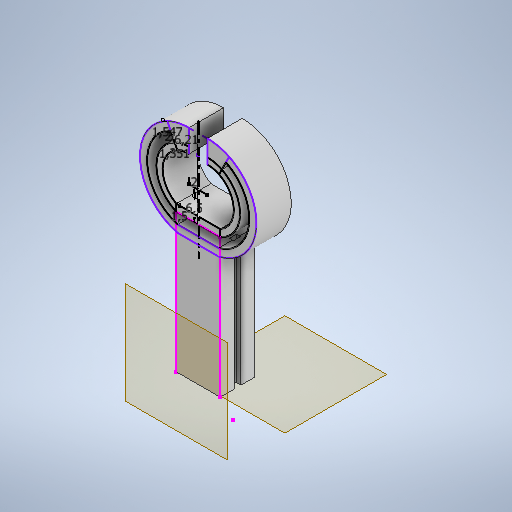
# Autodesk Inventor part: SlangHållare
Saved by Autodesk Inventor 2025.2 (Build 292293000, 293)
## iProperties
Created: 2025-01-28
Part Number: SlangHållare
Material: Generic
Document SubType Name: Modeling
Designer: 24oscnor
Density: 1 g/cm^3
Appearance: Default
Author: 24oscnor
Autodesk Inventor part; units mm, degrees
ref_plane "YZ Plane" through (0, 0, 0) normal (1, 0, 0) x (0, 1, 0)
ref_plane "XZ Plane" through (0, 0, 0) normal (0, 1, 0) x (-1, 0, 0)
ref_plane "XY Plane" through (0, 0, 0) normal (0, 0, 1) x (1, 0, 0)
ref_plane "Work Plane1" through (0, 3, 0) normal (0, 1, 0) x (1, 0, 0)
sketch "Sketch2" plane through (0, 3, 0) normal (0, 1, 0) x (1, 0, 0)
  line L0 (-11.25, -11.25) -> (-3.75, -11.25)
  line L1 (-3.75, -11.25) -> (-3.75, -3.75)
  line L2 (-3.75, -3.75) -> (-11.25, -3.75)
  line L3 (-11.25, -3.75) -> (-11.25, -11.25)
  line L4 (0, -15) -> (0, 0) projected
  line L5 (0, 0) -> (-15, 0) projected
  line L6 (-3.75, -11.25) -> (-2.75, -11.25)
  line L7 (-2.75, -11.25) -> (-2.75, -8.25)
  line L8 (-2.75, -8.25) -> (-3.75, -8.25)
  line L9 (-3.75, -8.25) -> (-3.75, -11.25)
  line L10 (-14.1659, -7.5) -> (-0.7229, -7.5) construction
  line L11 (-7.5, -11.25) -> (-7.5, -3.75) construction
  line L12 (-3.75, -3.75) -> (-2.75, -3.75)
  line L13 (-2.75, -3.75) -> (-2.75, -6.75)
  line L14 (-2.75, -6.75) -> (-3.75, -6.75)
  line L15 (-11.25, -11.25) -> (-12.25, -11.25)
  line L16 (-12.25, -11.25) -> (-12.25, -8.25)
  line L17 (-12.25, -8.25) -> (-11.25, -8.25)
  line L18 (-0.8341, -7.5) -> (-14.2771, -7.5) construction
  line L19 (-12.25, -3.75) -> (-12.25, -6.75)
  line L20 (-11.25, -3.75) -> (-12.25, -3.75)
  line L21 (-12.25, -6.75) -> (-11.25, -6.75)
  dimension "d4" = 7.5
  dimension "d5" = 7.5
  dimension "d6" = 3.75
  dimension "d7" = 3.75
  dimension "d8" = 3
  dimension "d9" = 1
  constraints: 40 end point, 11 symmetric about line, 4 parallel, 3 horizontal, 2 midpoint, 2 perpendicular
  measures "d4" distance between parallel lines of L3 L1
  measures "d5" distance between parallel lines of L2 L0
  measures "d6" distance between parallel lines of L4 L1
  measures "d7" distance between parallel lines of L5 L2
  measures "d8" distance of L6.end L7.end
  measures "d9" distance of L7.end L8.end
extrude "Extrusion2" add sketch "Sketch2" along normal blind 30
ref_plane "Work Plane2" through (-12.25, 3, 11.25) normal (0, 0, 1) x (1, 0, 0)
sketch "Sketch3" plane through (-12.25, 3, 11.25) normal (0, 0, 1) x (1, 0, 0)
  line L0 (0, 30) -> (9.5, 30) projected
  line L1 (9.5, 30) -> (0, 30) projected
  line L2 (4.75, 30) -> (4.75, 36.5)
  line L3 (4.75, 36.5) -> (2.75, 36.5)
  arc A0 (2.75, 43.5578) -> (0, 30) centre (2.75, 36.5) ccw
  line L4 (0, 0) -> (0, 30) projected
  line L5 (0, 30) -> (0, 31.5)
  arc A1 (0.23, 41.6198) -> (0, 31.5) centre (2.75, 36.5) ccw
  line L6 (9.5, 0) -> (9.5, 30) projected
  line L7 (9.5, 30) -> (9.5, 31.5)
  line L8 (0.23, 41.6198) -> (-0.3668, 42.8323)
  line L9 (-0.3668, 42.8323) -> (-1.25, 44.6267)
  arc A2 (-1.25, 44.6267) -> (0.3406, 27.7685) centre (2.75, 36.5) ccw
  arc A3 (3.75, 47.0578) -> (0.3417, 26.172) centre (2.75, 36.5) ccw
  line L10 (0, 30) -> (9.5, 30)
  line L11 (9.5, 31.5) -> (0, 31.5)
  line L12 (0.3406, 27.7685) -> (9.1594, 27.7685)
  line L13 (8.9409, 26.172) -> (0.3417, 26.172)
  line L14 (4.75, 36.5) -> (4.75, 49.394)
  line L15 (-1.25, 44.6267) -> (-1.9333, 46.0149)
  arc A4 (2.75, 42.2064) -> (0.23, 41.6198) centre (2.75, 36.5) ccw
  line L16 (2.75, 42.2064) -> (2.75, 47.105)
  line L17 (4.75, 49.394) -> (4.75, 23.6593)
  line L18 (4.75, 36.5) -> (6.75, 36.5)
  arc A5 (9.5, 30) -> (6.75, 43.5578) centre (6.75, 36.5) ccw
  line L19 (9.5, 30) -> (9.5, 31.5)
  arc A6 (9.5, 31.5) -> (9.27, 41.6198) centre (6.75, 36.5) ccw
  line L20 (9.27, 41.6198) -> (9.8668, 42.8323)
  line L21 (9.8668, 42.8323) -> (10.75, 44.6267)
  arc A7 (9.1594, 27.7685) -> (10.75, 44.6267) centre (6.75, 36.5) ccw
  arc A8 (9.1583, 26.172) -> (5.75, 47.0578) centre (6.75, 36.5) ccw
  line L22 (10.75, 44.6267) -> (11.4333, 46.0149)
  arc A9 (9.27, 41.6198) -> (6.75, 42.2064) centre (6.75, 36.5) ccw
  line L23 (6.75, 42.2064) -> (6.75, 47.105)
  point P0 (12.25, -3)
  point P1 (0, 27.8698)
  point P2 (4.75, 42.947)
  point P3 (9.5, 27.8698)
  point P4 (0, 26.2577)
  point P5 (9.5, 26.2577)
  dimension "d28" = 6.5
  dimension "d29" = 2
  dimension "d31" = 1.5
  dimension "d33" = 2
  dimension "d34" = 1.3514
  dimension "d59" = 26.207
  dimension "d60" = 1.5473
  constraints: 40 end point, 26 point on circle, 15 symmetric about line, 10 centre point, 10 coincident, 6 vertical, 3 perpendicular, 2 midpoint, 2 point on line, 1 horizontal, 5 other
  measures "d28" distance of L2.start L2.end
  measures "d29" distance of L2.end L3.end
  measures "d31" distance of L0.start L5.end
  measures "d33" distance of L8.end L9.end
  measures "d34" distance of L8.start L8.end
  measures "d59" angle of L14 L9
  measures "d60" distance of L9.end L15.end
extrude "Extrusion5" add sketch "Sketch3" against normal blind 7.5 contours L5 L11 L2 L0 | A0 L8 A1 L5 | L2 L11 L7 L0 | L9 L15 A3 L16 A0 | A0 L16 A4 L8 | L4 A3 L15 A2 | L7 A6 L20 A5 | A7 L22 A8 L6 | L20 A9 L23 A5 | A5 L23 A8 L22 L21
extrude "Extrusion6" cut sketch "Sketch3" against normal blind 7.5 contours L0 L17 L12 A2 L4 | L0 L6 A7 L12 L17
body "Solid1"
